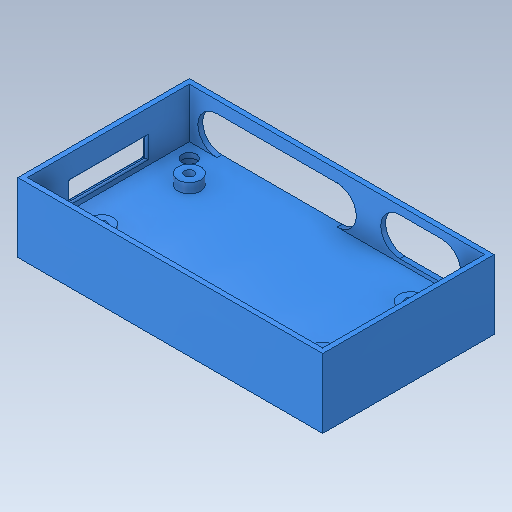
# Autodesk Inventor part: CaseBottomForPiZeroW
Saved by Autodesk Inventor 2021 (Build 250183000, 183)
## iProperties
Created: 2018-12-18
Part Number: CaseBottomForPiZeroW
Material: LCP Plastic
Document SubType Name: Modeling
Designer: steele
Density: 1.626 g/cm^3
Appearance: Cyan
PiZeroWLength: 2.559 in
PiZeroWWidth: 1.181 in
CaseLength: 3.150 in
CaseWidth: 1.772 in
CaseHeight: 0.515 in
PiZeroWMountingHole: 0.108 in
CaseWallThickness: 0.050 in
CaseFloorThickness: 0.200 in
PiZeroMoutingHolesLength: 2.283 in
PiZeroMountingHolesWidth: 0.906 in
PiZeroHoleSupport: 0.236 in
PiZeroWHoleHeight: 0.100 in
PiRibbonCableWidth: 0.787 in
PiRibbonCableThickness: 0.197 in
HdmiCenter: 0.748 in
MiniUsbCenter: 1.630 in
PowerCenter: 2.126 in
HdmiWidth: 1.102 in
MiniUsbWidth: 0.709 in
PowerWidth: 0.787 in
EndOfCaseToStartOfPiZero: 0.295 in
EyepieceOutsideDiameter: 1.250 in
EyepieceWallThickness: 0.075 in
EyepieceInnerDiameter: 1.100 in
PiRibbonCableHeightFromTp: 0.350 in
NutHeightPlusOffset: 0.073 in
NutWidthPlusOffset: 0.198 in
FilletForRibbonCable: 0.017 in
Author: steele
Autodesk Inventor part; units mm, degrees
ref_plane "YZ Plane" through (0, 0, 0) normal (1, 0, 0) x (0, 1, 0)
ref_plane "XZ Plane" through (0, 0, 0) normal (0, 1, 0) x (-1, 0, 0)
ref_plane "XY Plane" through (0, 0, 0) normal (0, 0, 1) x (1, 0, 0)
sketch "Sketch1" plane through (0, 0, 0) normal (0, 1, 0) x (-1, 0, 0)
  line L0 (40, 22.5) -> (-40, 22.5)
  line L1 (-40, 22.5) -> (-40, -22.5)
  line L2 (-40, -22.5) -> (40, -22.5)
  line L3 (40, -22.5) -> (40, 22.5)
  line L4 (40, 22.5) -> (-40, -22.5) construction
  line L5 (-40, 22.5) -> (40, -22.5) construction
  point P0 (0, 0)
  dimension "d0" = 80
  dimension "d1" = 45
  constraints: 12 end point, 2 midpoint, 2 parallel, 1 horizontal, 1 perpendicular
  measures "d0" distance of L1.end L2.end
  measures "d1" distance of L2.end L0.start
extrude "Extrusion1" add sketch "Sketch1" against normal blind 5.08
sketch "Sketch2" plane through (0, 0, 0) normal (0, 1, 0) x (1, 0, 0)
  line L0 (40, -22.5) -> (-40, -22.5) projected
  line L1 (-40, 22.5) -> (40, 22.5) projected
  line L2 (-40, -22.5) -> (40, -22.5)
  line L3 (40, -22.5) -> (40, 22.5)
  line L4 (40, 22.5) -> (-40, 22.5)
  line L5 (-40, 22.5) -> (-40, -22.5)
  line L6 (-38.73, -21.23) -> (38.73, -21.23)
  line L7 (38.73, -21.23) -> (38.73, 21.23)
  line L8 (38.73, 21.23) -> (-38.73, 21.23)
  line L9 (-38.73, 21.23) -> (-38.73, -21.23)
  line L10 (-38.73, -21.23) -> (38.73, 21.23) construction
  line L11 (38.73, -21.23) -> (-38.73, 21.23) construction
  point P0 (0, 0)
  dimension "d4" = 1.27
  dimension "d5" = 1.27
  constraints: 20 end point, 4 parallel, 2 horizontal, 2 midpoint, 2 perpendicular
  measures "d4" distance between parallel lines of L9 L5
  measures "d5" distance between parallel lines of L0 L6
extrude "Extrusion2" add sketch "Sketch2" along normal blind 13.08
sketch "Sketch3" plane through (0, 0, 0) normal (0, 1, 0) x (1, 0, 0)
  line L0 (-29, -11.5) -> (29, -11.5) construction
  line L1 (29, -11.5) -> (29, 11.5) construction
  line L2 (29, 11.5) -> (-29, 11.5) construction
  line L3 (-29, 11.5) -> (-29, -11.5) construction
  line L4 (-29, -11.5) -> (29, 11.5) construction
  line L5 (29, -11.5) -> (-29, 11.5) construction
  circle A0 centre (-29, -11.5) radius 3
  circle A1 centre (29, -11.5) radius 3
  circle A2 centre (-29, 11.5) radius 3
  circle A3 centre (29, 11.5) radius 3
  point P0 (0, 0)
  dimension "d8" = 23
  dimension "d9" = 58
  dimension "d19" = 58
  dimension "d22" = 23
  dimension "d25" = 6
  constraints: 12 end point, 4 centre point, 2 coincident, 2 horizontal, 2 midpoint, 2 parallel, 1 perpendicular, 1 vertical, 6 other
  measures "d8" distance of L2.end L0.start
  measures "d9" distance of L1.end L2.end
  measures "d19" distance of A0.centre A1.centre
  measures "d22" distance of A0.centre A2.centre
  measures "d25" diameter of A0
extrude "Extrusion3" add sketch "Sketch3" along normal blind 2.54
sketch "Sketch5" plane through (-40, -5.08, -22.5) normal (-1, 0, 0) x (0, 0, 1)
  line L0 (43.73, 18.16) -> (1.27, 18.16) construction
  line L1 (22.5, 18.16) -> (22.5, 5.08) construction
  line L2 (45, 18.16) -> (45, 0) construction
  line L3 (45, 9.27) -> (0, 9.27) construction
  line L4 (0, 0) -> (0, 18.16) construction
  line L5 (12.5, 11.77) -> (32.5, 11.77)
  line L6 (32.5, 11.77) -> (32.5, 6.77)
  line L7 (32.5, 6.77) -> (12.5, 6.77)
  line L8 (12.5, 6.77) -> (12.5, 11.77)
  line L9 (12.5, 11.77) -> (32.5, 6.77) construction
  line L10 (32.5, 11.77) -> (12.5, 6.77) construction
  line L11 (0, 18.16) -> (45, 18.16) projected
  point P0 (22.5, 9.27)
  dimension "d35" = 20
  dimension "d36" = 5
  dimension "d99" = 8.89
  constraints: 16 end point, 4 midpoint, 3 parallel, 2 point on line, 1 horizontal, 1 perpendicular, 1 vertical
  measures "d35" distance of L5.start L5.end
  measures "d36" distance of L7.end L5.start
  measures "d99" distance from line of L0 point (22.5, 9.27)
extrude "ExtrusionForRibbonCableHole" cut sketch "Sketch5" against normal up to next
sketch "Sketch6" plane through (40, -5.08, -22.5) normal (0, 0, -1) x (-1, 0, 0)
  line L0 (0, 18.16) -> (80, 18.16) construction
  line L1 (0, 0) -> (0, 18.16) construction
  line L2 (80, 18.16) -> (80, 0) construction
  line L3 (12.5, 11.08) -> (40.5, 11.08) construction
  line L4 (12.5, 6.08) -> (23.5, 6.08)
  line L5 (23.5, 16.08) -> (12.5, 16.08)
  arc A0 (12.5, 16.08) -> (12.5, 6.08) centre (12.5, 11.08) ccw
  arc A1 (23.5, 6.08) -> (23.5, 16.08) centre (23.5, 11.08) ccw
  line L6 (39.9, 10.08) -> (57.9, 10.08) construction
  line L7 (39.9, 5.08) -> (57.9, 5.08)
  line L8 (57.9, 15.08) -> (39.9, 15.08)
  arc A2 (39.9, 15.08) -> (39.9, 5.08) centre (39.9, 10.08) ccw
  arc A3 (57.9, 5.08) -> (57.9, 15.08) centre (57.9, 10.08) ccw
  line L9 (51.5, 10.08) -> (71.5, 10.08) construction
  line L10 (51.5, 5.08) -> (71.5, 5.08)
  line L11 (71.5, 15.08) -> (51.5, 15.08)
  arc A4 (51.5, 15.08) -> (51.5, 5.08) centre (51.5, 10.08) ccw
  arc A5 (71.5, 5.08) -> (71.5, 15.08) centre (71.5, 10.08) ccw
  line L12 (1.27, 5.08) -> (78.73, 5.08) projected
  point P0 (40, 5.08)
  point P1 (26.5, 11.08)
  point P2 (48.9, 10.08)
  point P3 (61.5, 10.08)
  dimension "d39" = 10
  dimension "d40" = 26.5
  dimension "d41" = 28
  dimension "d42" = 48.9
  dimension "d43" = 10
  dimension "d44" = 18
  dimension "d45" = 10
  dimension "d46" = 20
  dimension "d47" = 61.5
  dimension "d50" = 6
  dimension "d51" = 5
  dimension "d52" = 5
  constraints: 23 end point, 12 point on circle, 12 tangent, 6 centre point, 3 midpoint, 3 parallel
  measures "d39" distance between parallel lines of L5 L4
  measures "d40" distance from line of point (26.5, 11.08) L1
  measures "d41" distance of L3.end L3.start
  measures "d42" distance from line of point (48.9, 10.08) L1
  measures "d43" distance between parallel lines of L8 L7
  measures "d44" distance of L6.end L6.start
  measures "d45" distance between parallel lines of L10 L11
  measures "d46" distance of L9.start L9.end
  measures "d47" distance from line of point (61.5, 10.08) L1
  measures "d50" distance from line of L12 point (26.5, 11.08)
  measures "d51" distance from line of L12 point (48.9, 10.08)
  measures "d52" distance from line of L12 point (61.5, 10.08)
extrude "ExtrusionForSideHoles" cut sketch "Sketch6" against normal blind 1.27
fillet "FilletForRibbonCable" radius 0.4233 8 edges at (-40, 1.69, 0) (-40, 4.19, -10) (-40, 6.69, 0) (-40, 4.19, 10) (-38.73, 4.19, -10) (-38.73, 6.69, 0) (-38.73, 1.69, 0) (-38.73, 4.19, 10)
sketch "Sketch22" plane through (0, -5.08, 0) normal (0, -1, 0) x (1, 0, 0)
  point P0 (34.92, -17.42)
  point P1 (34.92, 17.42)
  point P2 (-34.92, 17.42)
  point P3 (-34.92, -17.42)
hole "Hole12" at (34.92, -5.08, -17.42) at (34.92, -5.08, 17.42) at (-34.92, -5.08, 17.42) at (-34.92, -5.08, -17.42) direction (0, 1, 0) diameter 3.7973 depth 5.08
sketch "Sketch23" plane through (0, -5.08, 0) normal (0, -1, 0) x (1, 0, 0)
  circle A0 centre (-34.92, 17.42) radius 1.8986 projected
  circle A1 centre (34.92, 17.42) radius 1.8986 projected
  circle A2 centre (34.92, -17.42) radius 1.8986 projected
  circle A3 centre (-34.92, -17.42) radius 1.8986 projected
  point P0 (0, 0)
  constraints: 4 coincident
hole "Hole13" at (-34.92, -5.08, 17.42) at (34.92, -5.08, 17.42) at (34.92, -5.08, -17.42) at (-34.92, -5.08, -17.42) direction (0, 1, 0) diameter 4.8514 depth 3.81
sketch "Sketch25" plane through (0, -5.08, 0) normal (0, -1, 0) x (1, 0, 0)
  circle A0 centre (29, 11.5) radius 3 projected
  circle A1 centre (29, -11.5) radius 3 projected
  circle A2 centre (-29, -11.5) radius 3 projected
  circle A3 centre (-29, 11.5) radius 3 projected
  point P0 (0, 0)
  constraints: 4 coincident
hole "Hole16" at (29, -5.08, 11.5) at (29, -5.08, -11.5) at (-29, -5.08, -11.5) at (-29, -5.08, 11.5) direction (0, 1, 0) diameter 2.4384 end through all counterbore diameter 3.2639 counterbore depth 3.9878
equation "\"d0\" = CaseLength"
equation "\"d1\" = CaseWidth"
equation "\"d2\" = CaseFloorThickness"
equation "\"d4\" = CaseWallThickness"
equation "\"d5\" = CaseWallThickness"
equation "\"d6\" = CaseHeight"
equation "\"d8\" = PiZeroMountingHolesWidth"
equation "\"d9\" = PiZeroMoutingHolesLength"
equation "\"d19\" = PiZeroMoutingHolesLength"
equation "\"d22\" = PiZeroMountingHolesWidth"
equation "\"d25\" = PiZeroHoleSupport"
equation "\"d26\" = PiZeroWHoleHeight"
equation "\"d35\" = PiRibbonCableWidth"
equation "\"d36\" = PiRibbonCableThickness"
equation "\"d99\" = PiRibbonCableHeightFromTp"
equation "\"d39\" = HdmiHeight"
equation "\"d40\" = EndOfCaseToStartOfPiZero + HdmiCenter"
equation "\"d41\" = HdmiWidth"
equation "\"d42\" = EndOfCaseToStartOfPiZero + MiniUsbCenter"
equation "\"d43\" = MiniUsbHeight"
equation "\"d44\" = MiniUsbWidth"
equation "\"d45\" = PowerHeight"
equation "\"d46\" = PowerWidth"
equation "\"d47\" = EndOfCaseToStartOfPiZero + PowerCenter"
equation "\"d50\" = HdmiHightAboveBottom"
equation "\"d51\" = MiniUsbHeightAboveBottom"
equation "\"d52\" = PowerHeightAboveBottom"
equation "\"d97\" = CaseWallThickness"
equation "\"d100\" = FilletForRibbonCable"
equation "\"PiZeroWLength\" = 65"
equation "\"PiZeroWWidth\" = 30"
equation "\"CaseLength\" = PiZeroWLength + 2 * EndOfCaseToStartOfPiZero"
equation "\"CaseWidth\" = PiZeroWWidth + 2 * EndOfCaseToStartOfPiZero"
equation "\"PiZeroWMountingHole\" = 2.75"
equation "\"CaseWallThickness\" = 1.27"
equation "\"CaseFloorThickness\" = 5.08"
equation "\"PiZeroMoutingHolesLength\" = 58"
equation "\"PiZeroMountingHolesWidth\" = 23"
equation "\"PiZeroHoleSupport\" = 6"
equation "\"PiZeroWHoleHeight\" = 2.54"
equation "\"PiRibbonCableWidth\" = 20"
equation "\"PiRibbonCableThickness\" = 5"
equation "\"HdmiCenter\" = 19"
equation "\"MiniUsbCenter\" = 41.4"
equation "\"PowerCenter\" = 54"
equation "\"HdmiWidth\" = 28"
equation "\"MiniUsbWidth\" = 18"
equation "\"PowerWidth\" = 20"
equation "\"EndOfCaseToStartOfPiZero\" = 7.5"
equation "\"EyepieceOutsideDiameter\" = 31.75"
equation "\"EyepieceWallThickness\" = 1.905"
equation "\"EyepieceInnerDiameter\" = EyepieceOutsideDiameter - 2 * EyepieceWallThickness"
equation "\"HeightOfConnectorHolesAboveBottom\" = 6"
equation "\"HdmiHeight\" = 10"
equation "\"MiniUsbHeight\" = 10"
equation "\"PowerHeight\" = 10"
equation "\"HdmiHightAboveBottom\" = 6"
equation "\"MiniUsbHeightAboveBottom\" = 5"
equation "\"PowerHeightAboveBottom\" = 5"
equation "\"PiRibbonCableHeightFromTp\" = 8.89"
equation "\"NutHeightPlusOffset\" = 1.8415"
equation "\"NutWidthPlusOffset\" = 5.0165"
equation "\"FilletForRibbonCable\" = 0.333333 * CaseWallThickness"
equation "\"CaseHeight\" = 13.08"
body "Solid1"
